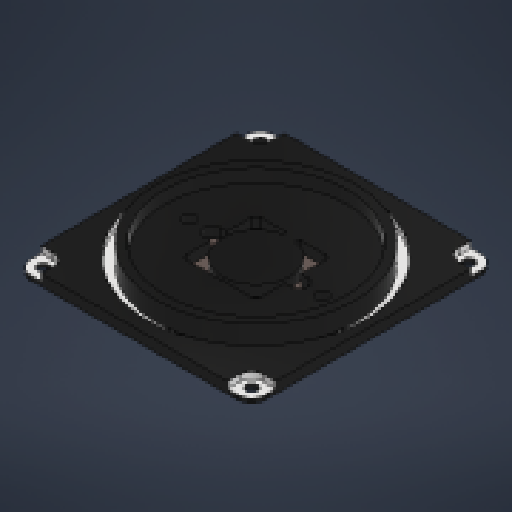
# Autodesk Inventor part: Camera_Mount
Saved by Autodesk Inventor 2024.2 (Build 282272000, 272)
## iProperties
Created: 2024-01-10
Part Number: Camera_Mount
Material: 一般
Document SubType Name: Modeling
Designer: Hanaoka
Density: 1 g/cm^3
Appearance: 既定
Author: Hanaoka
Autodesk Inventor part; units mm, degrees
ref_plane "YZ Plane" through (0, 0, 0) normal (1, 0, 0) x (0, 1, 0)
ref_plane "XZ Plane" through (0, 0, 0) normal (0, 1, 0) x (-1, 0, 0)
ref_plane "XY Plane" through (0, 0, 0) normal (0, 0, 1) x (1, 0, 0)
ref_plane "作業平面1" through (56.3598, -66.4332, -0.2999) normal (0, 1, 0) x (1, 0, 0)
sketch "スケッチ1" plane through (56.3598, -66.4332, -0.2999) normal (0, 1, 0) x (1, 0, 0)
  line L0 (9.655, 16.755) -> (9.655, 15.8775) projected
  arc A0 (6.855, 15.8775) -> (9.655, 15.8775) centre (8.255, 8.255) ccw projected
  line L1 (6.855, 15.8775) -> (6.855, 16.755) projected
  line L2 (6.855, 16.755) -> (0.755, 16.755) projected
  arc A1 (0.755, 16.755) -> (-0.245, 15.755) centre (0.755, 15.755) ccw projected
  line L3 (-0.245, 15.755) -> (-0.245, 10.155) projected
  line L4 (-0.245, 10.155) -> (-1.745, 10.155) projected
  arc A2 (-1.745, 10.155) -> (-1.745, 6.355) centre (-1.745, 8.255) ccw projected
  line L5 (-1.745, 6.355) -> (-0.245, 6.355) projected
  line L6 (-0.245, 6.355) -> (-0.245, 0.755) projected
  arc A3 (-0.245, 0.755) -> (0.755, -0.245) centre (0.755, 0.755) ccw projected
  line L7 (0.755, -0.245) -> (15.755, -0.245) projected
  arc A4 (15.755, -0.245) -> (16.755, 0.755) centre (15.755, 0.755) ccw projected
  line L8 (16.755, 0.755) -> (16.755, 6.355) projected
  line L9 (16.755, 6.355) -> (18.255, 6.355) projected
  arc A5 (18.255, 6.355) -> (18.255, 10.155) centre (18.255, 8.255) ccw projected
  line L10 (18.255, 10.155) -> (16.755, 10.155) projected
  line L11 (16.755, 10.155) -> (16.755, 15.755) projected
  arc A6 (16.755, 15.755) -> (15.755, 16.755) centre (15.755, 15.755) ccw projected
  line L12 (15.755, 16.755) -> (9.655, 16.755) projected
  circle A7 centre (-1.745, 8.255) radius 0.9 projected
  circle A8 centre (18.255, 8.255) radius 0.9 projected
  circle A9 centre (-6.985, 8.255) radius 1.5 projected
  circle A10 centre (23.495, 8.255) radius 1.5 projected
  line L13 (-15.745, -19.745) -> (32.255, -19.745)
  line L14 (35.255, -16.745) -> (35.255, 33.255)
  line L15 (32.255, 36.255) -> (-15.745, 36.255)
  line L16 (-18.745, 33.255) -> (-18.745, -16.745)
  line L17 (-18.745, -19.745) -> (35.255, 36.255) construction
  line L18 (35.255, -19.745) -> (-18.745, 36.255) construction
  line L19 (8.255, 36.255) -> (8.255, -19.745) construction
  line L20 (-18.745, 8.255) -> (35.255, 8.255) construction
  arc A11 (-15.745, 36.255) -> (-18.745, 33.255) centre (-15.745, 33.255) ccw
  arc A12 (35.255, 33.255) -> (32.255, 36.255) centre (32.255, 33.255) ccw
  arc A13 (32.255, -19.745) -> (35.255, -16.745) centre (32.255, -16.745) ccw
  arc A14 (-18.745, -16.745) -> (-15.745, -19.745) centre (-15.745, -16.745) ccw
  circle A15 centre (-15.745, 33.255) radius 1.3
  circle A16 centre (32.255, 33.255) radius 1.3
  circle A17 centre (-15.745, -16.745) radius 1.3
  circle A18 centre (32.255, -16.745) radius 1.3
  circle A19 centre (8.255, 8.255) radius 25
  line L21 (32.255, -16.745) -> (-15.745, -16.745) construction
  line L22 (-15.745, -16.745) -> (-15.745, 33.255) construction
  line L23 (-15.745, 33.255) -> (32.255, 33.255) construction
  line L24 (32.255, 33.255) -> (32.255, -16.745) construction
  line L25 (32.255, -16.745) -> (-15.745, 33.255) construction
  line L26 (-15.745, -16.745) -> (32.255, 33.255) construction
  point P0 (-56.3598, -0.2999)
  dimension "d0" = 3
  dimension "d2" = 54
  dimension "d3" = 2.6
  dimension "d4" = 50
  dimension "d7" = 48
  dimension "d8" = 50
  dimension "d9" = 56
  constraints: 28 end point, 10 midpoint, 9 centre point, 8 point on circle, 8 point on line, 8 tangent, 6 equal radius, 5 coincident, 4 parallel, 2 horizontal, 2 perpendicular
  measures "d0" radius of A11
  measures "d2" distance between parallel lines of L14 L16
  measures "d3" diameter of A15
  measures "d4" diameter of A19
  measures "d7" distance of L22.end L23.end
  measures "d8" distance of L23.end L21.start
  measures "d9" distance between parallel lines of L13 L15
extrude "押し出し1" add sketch "スケッチ1" along normal blind 2.5 contours A14 L16 A11 L15 A12 L14 A13 L13 | A19
sketch "スケッチ2" plane through (56.3598, -63.9332, -0.2999) normal (0, 1, 0) x (1, 0, 0)
  arc A0 (32.255, -19.745) -> (35.255, -16.745) centre (32.255, -16.745) ccw projected
  line L0 (35.255, -16.745) -> (35.255, 33.255) projected
  arc A1 (35.255, 33.255) -> (32.255, 36.255) centre (32.255, 33.255) ccw projected
  line L1 (32.255, 36.255) -> (-15.745, 36.255) projected
  arc A2 (-15.745, 36.255) -> (-18.745, 33.255) centre (-15.745, 33.255) ccw projected
  line L2 (-18.745, 33.255) -> (-18.745, -16.745) projected
  arc A3 (-18.745, -16.745) -> (-15.745, -19.745) centre (-15.745, -16.745) ccw projected
  line L3 (-15.745, -19.745) -> (32.255, -19.745) projected
  arc A4 (6.855, 15.8775) -> (9.655, 15.8775) centre (8.255, 8.255) ccw projected
  line L4 (9.655, 15.8775) -> (9.655, 16.755) projected
  line L5 (9.655, 16.755) -> (15.755, 16.755) projected
  arc A5 (16.755, 15.755) -> (15.755, 16.755) centre (15.755, 15.755) ccw projected
  line L6 (16.755, 15.755) -> (16.755, 10.155) projected
  line L7 (16.755, 10.155) -> (18.255, 10.155) projected
  arc A6 (18.255, 6.355) -> (18.255, 10.155) centre (18.255, 8.255) ccw projected
  line L8 (18.255, 6.355) -> (16.755, 6.355) projected
  line L9 (16.755, 6.355) -> (16.755, 0.755) projected
  arc A7 (15.755, -0.245) -> (16.755, 0.755) centre (15.755, 0.755) ccw projected
  line L10 (15.755, -0.245) -> (0.755, -0.245) projected
  arc A8 (-0.245, 0.755) -> (0.755, -0.245) centre (0.755, 0.755) ccw projected
  line L11 (-0.245, 0.755) -> (-0.245, 6.355) projected
  line L12 (-0.245, 6.355) -> (-1.745, 6.355) projected
  arc A9 (-1.745, 10.155) -> (-1.745, 6.355) centre (-1.745, 8.255) ccw projected
  line L13 (-1.745, 10.155) -> (-0.245, 10.155) projected
  line L14 (-0.245, 10.155) -> (-0.245, 15.755) projected
  arc A10 (0.755, 16.755) -> (-0.245, 15.755) centre (0.755, 15.755) ccw projected
  line L15 (0.755, 16.755) -> (6.855, 16.755) projected
  line L16 (6.855, 16.755) -> (6.855, 15.8775) projected
  circle A11 centre (-6.985, 8.255) radius 1.5 projected
  circle A12 centre (23.495, 8.255) radius 1.5 projected
  circle A13 centre (32.255, -16.745) radius 1.3 projected
  circle A14 centre (-15.745, -16.745) radius 1.3 projected
  circle A15 centre (32.255, 33.255) radius 1.3 projected
  circle A16 centre (-15.745, 33.255) radius 1.3 projected
  circle A17 centre (8.255, 8.255) radius 23
  circle A18 centre (8.255, 8.255) radius 21
  circle A19 centre (8.255, 8.255) radius 25
  arc A20 (-13.245, -16.745) -> (-15.745, -14.245) centre (-15.745, -16.745) ccw
  arc A21 (-15.745, 30.755) -> (-13.245, 33.255) centre (-15.745, 33.255) ccw
  arc A22 (32.255, -14.245) -> (29.755, -16.745) centre (32.255, -16.745) ccw
  arc A23 (29.755, 33.255) -> (32.255, 30.755) centre (32.255, 33.255) ccw
  line L17 (-15.745, -14.245) -> (-18.745, -14.245)
  line L18 (-13.245, -16.745) -> (-13.245, -19.745)
  line L19 (-15.745, 30.755) -> (-18.745, 30.755)
  line L20 (-13.245, 33.255) -> (-13.245, 36.255)
  line L21 (29.755, 33.255) -> (29.755, 36.255)
  line L22 (32.255, 30.755) -> (35.255, 30.755)
  line L23 (32.255, -14.245) -> (35.255, -14.245)
  line L24 (29.755, -16.745) -> (29.755, -19.745)
  line L25 (-18.745, 33.255) -> (-18.745, -16.745) projected
  line L26 (-15.745, -19.745) -> (32.255, -19.745) projected
  line L27 (32.255, 36.255) -> (-15.745, 36.255) projected
  line L28 (35.255, -16.745) -> (35.255, 33.255) projected
  point P0 (-56.3598, -0.2999)
  dimension "d10" = 46
  dimension "d11" = 2
  dimension "d14" = 50
  dimension "d15" = 2.5
  constraints: 16 end point, 9 perpendicular, 9 point on line, 8 point on circle, 8 tangent, 7 centre point, 7 coincident, 3 equal radius, 1 horizontal, 1 vertical
  measures "d10" diameter of A17
  measures "d11" radial gap between concentric circles of A17 A18
  measures "d14" diameter of A19
  measures "d15" radius of A20
extrude "押し出し2" add sketch "スケッチ2" along normal blind 3 contours A17
extrude "押し出し4" cut sketch "スケッチ2" against normal blind 1 contours L3 L24 A22 L23 L0 A0 | L3 A3 L2 L17 A20 L18 | L22 A23 L21 L1 A1 L0 | L2 A2 L1 L20 A21 L19 | A19
